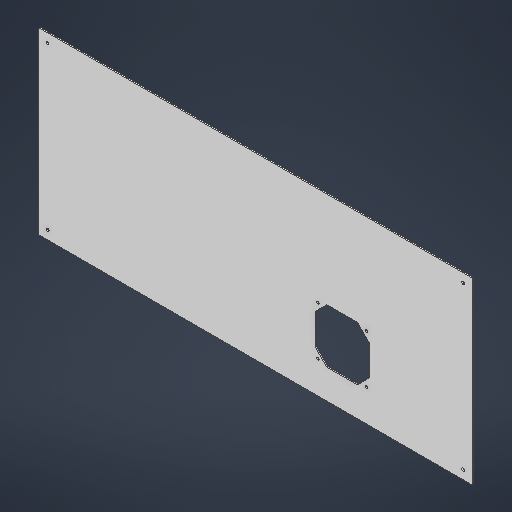
# Autodesk Inventor part: PlaqueVentilo
Saved by Autodesk Inventor 2026.2 (Build 302298010, 298A)
## iProperties
Created: 2026-05-13
Part Number: PlaqueVentilo
Material: Générique
Document SubType Name: Modeling
Designer: romai
Density: 1 g/cm^3
Appearance: Par défaut
Author: romai
Autodesk Inventor part; units mm, degrees
ref_plane "YZ Plane" through (0, 0, 0) normal (1, 0, 0) x (0, 1, 0)
ref_plane "XZ Plane" through (0, 0, 0) normal (0, 1, 0) x (-1, 0, 0)
ref_plane "XY Plane" through (0, 0, 0) normal (0, 0, 1) x (1, 0, 0)
sketch "Esquisse1" plane through (0, 0, 0) normal (0, 0, 1) x (1, 0, 0)
  line L0 (-368.5, -152.5) -> (368.5, -152.5)
  line L1 (368.5, -152.5) -> (368.5, 152.5)
  line L2 (368.5, 152.5) -> (-368.5, 152.5)
  line L3 (-368.5, 152.5) -> (-368.5, -152.5)
  line L4 (-368.5, -152.5) -> (368.5, 152.5) construction
  line L5 (-356, -140) -> (356, -140)
  line L6 (356, -140) -> (356, 140)
  line L7 (356, 140) -> (-356, 140)
  line L8 (-356, 140) -> (-356, -140)
  line L9 (-356, -140) -> (356, 140) construction
  circle A0 centre (-353.5, 137.5) radius 2.5
  circle A1 centre (-353.5, -137.5) radius 2.5
  circle A2 centre (353.5, -137.5) radius 2.5
  circle A3 centre (353.5, 137.5) radius 2.5
  line L10 (121.5, -10.5) -> (173.5, -10.5)
  line L11 (193.5, -30.5) -> (193.5, -82.5)
  line L12 (173.5, -102.5) -> (121.5, -102.5)
  line L13 (101.5, -82.5) -> (101.5, -30.5)
  line L14 (101.5, -10.5) -> (193.5, -102.5) construction
  line L15 (193.5, -10.5) -> (101.5, -102.5) construction
  line L16 (121.5, -10.5) -> (101.5, -30.5)
  line L17 (101.5, -82.5) -> (121.5, -102.5)
  line L18 (173.5, -102.5) -> (193.5, -82.5)
  line L19 (193.5, -30.5) -> (173.5, -10.5)
  circle A4 centre (106.25, -15.25) radius 2.2
  circle A5 centre (188.75, -15.25) radius 2.2
  circle A6 centre (188.75, -97.75) radius 2.2
  circle A7 centre (106.25, -97.75) radius 2.2
  point P0 (0, 0)
  point P1 (-356, -137.5)
  point P2 (-353.5, -140)
  point P3 (353.5, -140)
  point P4 (356, -137.5)
  point P5 (356, 137.5)
  point P6 (353.5, 140)
  point P7 (-356, 137.5)
  point P8 (-353.5, 140)
  point P9 (147.5, -56.5)
  dimension "d0" = 737
  dimension "d1" = 305
  dimension "d2" = 12.5
  dimension "d3" = 12.5
  dimension "d4" = 5
  dimension "d7" = 5
  dimension "d8" = 5
  dimension "d9" = 5
  dimension "d36" = 92
  dimension "d37" = 92
  dimension "d38" = 50
  dimension "d39" = 175
  dimension "d48" = 20
  dimension "d49" = 20
  dimension "d50" = 20
  dimension "d51" = 20
  dimension "d52" = 20
  dimension "d53" = 20
  dimension "d54" = 20
  dimension "d55" = 20
  dimension "d57" = 4.4
  dimension "d58" = 4.4
  dimension "d59" = 4.4
  dimension "d60" = 4.4
  dimension "d61" = 4.75
  dimension "d62" = 4.75
  constraints: 40 end point, 19 point on line, 8 centre point, 8 tangent, 6 parallel, 4 midpoint, 3 horizontal, 3 perpendicular
  measures "d0" distance of L2.end L1.end
  measures "d1" distance of L1.end L0.end
  measures "d2" distance between parallel lines of L2 L7
  measures "d3" distance between parallel lines of L1 L6
  measures "d4" diameter of A0
  measures "d7" diameter of A1
  measures "d8" diameter of A2
  measures "d9" diameter of A3
  measures "d36" distance of L14.end L15.end
  measures "d37" distance of L15.start L14.end
  measures "d38" distance between parallel lines of L0 L12
  measures "d39" distance between parallel lines of L1 L11
  measures "d48" distance of L10.start point (101.5, -10.5)
  measures "d49" distance of L13.end point (101.5, -10.5)
  measures "d50" distance of L13.start point (101.5, -102.5)
  measures "d51" distance of L12.end point (101.5, -102.5)
  measures "d52" distance of L12.start point (193.5, -102.5)
  measures "d53" distance of L11.end point (193.5, -102.5)
  measures "d54" distance of L11.start point (193.5, -10.5)
  measures "d55" distance of L10.end point (193.5, -10.5)
  measures "d57" diameter of A4
  measures "d58" diameter of A5
  measures "d59" diameter of A6
  measures "d60" diameter of A7
  measures "d61" horizontal distance of L14.start A4.centre
  measures "d62" horizontal distance of L14.start A4.centre
extrude "Extrusion1" add sketch "Esquisse1" along normal blind 2 contours L3 L2 L1 L0 | L8 A1 L5 | A1 L8 A0 L7 A3 L6 A2 L5 | A2 L6 L5 | L8 L7 A0 | A3 L7 L6
equation "\"d49\" = d48"
equation "\"d50\" = d48"
equation "\"d51\" = d50"
equation "\"d52\" = d48"
equation "\"d53\" = d52"
equation "\"d54\" = d48"
equation "\"d55\" = d54"
